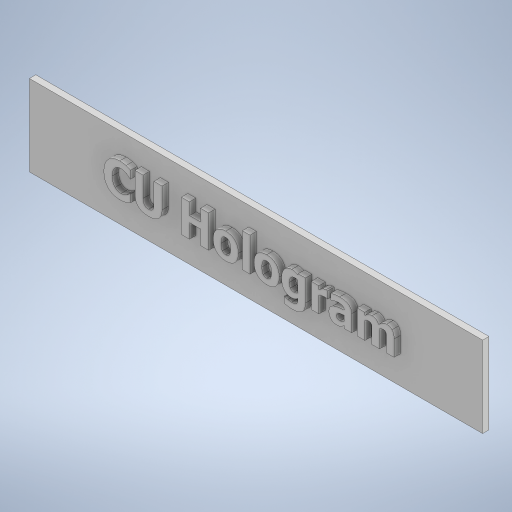
# Autodesk Inventor part: Apple iPad 2022 Hologram
Saved by Autodesk Inventor 2024 (Build 280153000, 153)
## iProperties
Created: 2024-02-23
Part Number: Apple iPad 2022 Hologram
Material: Generic
Document SubType Name: Modeling
Designer: littl
Density: 1 g/cm^3
Appearance: Default
Author: littl
Autodesk Inventor part; units mm, degrees
ref_plane "YZ Plane" through (0, 0, 0) normal (1, 0, 0) x (0, 1, 0)
ref_plane "Work Plane4" through (-177.8, 25.4, 133.35) normal (0, 0, 1) x (1, 0, 0)
sketch "Sketch7" plane through (-177.8, 25.4, 133.35) normal (0, 0, 1) x (1, 0, 0)
  line L0 (355.6, 0) -> (355.6, 12.7)
  line L1 (355.6, 12.7) -> (0, 12.7)
  line L2 (0, 12.7) -> (0, 0)
  line L3 (50.8, -25.4) -> (304.8, -25.4) projected
  line L4 (50.8, -25.4) -> (304.8, -25.4)
  line L5 (304.8, -50.8) -> (50.8, -50.8)
  line L6 (0, 12.7) -> (355.6, 12.7)
  line L7 (355.6, 12.7) -> (355.6, -50.8)
  line L8 (355.6, -50.8) -> (0, -50.8)
  line L9 (0, -50.8) -> (0, 12.7)
  point P0 (177.8, -25.4)
  point P1 (50.8, -50.8)
  dimension "d36" = 12.7
  dimension "d37" = 25.4
  constraints: 18 end point, 5 equal length, 1 horizontal, 1 perpendicular, 1 point on line
  measures "d36" distance of L0.end L0.start
  measures "d37" distance of L3.end L5.start
extrude "Decoration Plate" add sketch "Sketch7" along normal blind 5
ref_plane "Work Plane3" through (-177.8, 25.4, 138.35) normal (0, 0, 1) x (1, 0, 0)
sketch "Sketch8" plane through (-177.8, 25.4, 138.35) normal (0, 0, 1) x (1, 0, 0)
  line L0 (0, 12.7) -> (355.6, 12.7) construction
  line L1 (355.6, 12.7) -> (355.6, -50.8) construction
  line L2 (355.6, -50.8) -> (0, -50.8) construction
  line L3 (0, -50.8) -> (0, 12.7) construction
  line L4 (355.6, -50.8) -> (355.6, 12.7) projected
  line L5 (0, 12.7) -> (0, -50.8) projected
  line L6 (355.6, 12.7) -> (0, 12.7) projected
  line L7 (0, -50.8) -> (355.6, -50.8) projected
  spline S0 degree 2 poles (75.8604, -29.2079) (70.1382, -29.2079) (63.428, -22.2919) (63.428, -16.0345) knots 0 0 0 1 2 2 2
  spline S1 degree 2 poles (63.428, -16.0345) (63.428, -10.0036) (70.1588, -2.8199) (75.881, -2.8199) knots 0 0 0 1 2 2 2
  spline S2 degree 2 poles (75.881, -2.8199) (77.3836, -2.8199) (79.8124, -3.1699) (80.9239, -3.458) knots 0 0 0 1 2 2 2
  spline S3 degree 2 poles (80.9239, -3.458) (81.7884, -3.7256) (83.8262, -4.6107) (84.4643, -4.94) knots 0 0 0 1 2 2 2
  line L8 (84.4643, -4.94) -> (84.4643, -10.9916)
  line L9 (84.4643, -10.9916) -> (83.8262, -10.9916)
  spline S4 degree 2 poles (83.8262, -10.9916) (83.3528, -10.5799) (81.9531, -9.4272) (81.068, -8.8921) knots 0 0 0 1 2 2 2
  spline S5 degree 2 poles (81.068, -8.8921) (80.1829, -8.3363) (78.0628, -7.5747) (76.8896, -7.5747) knots 0 0 0 1 2 2 2
  spline S6 degree 2 poles (76.8896, -7.5747) (75.5105, -7.5747) (73.2257, -8.4392) (72.1759, -9.5301) knots 0 0 0 1 2 2 2
  spline S7 degree 2 poles (72.1759, -9.5301) (71.2291, -10.4976) (70.0147, -13.8115) (70.0147, -16.0551) knots 0 0 0 1 2 2 2
  spline S8 degree 2 poles (70.0147, -16.0551) (70.0147, -18.4222) (71.2703, -21.6538) (72.2994, -22.6418) knots 0 0 0 1 2 2 2
  spline S9 degree 2 poles (72.2994, -22.6418) (73.2874, -23.6092) (75.7163, -24.4532) (76.9307, -24.4532) knots 0 0 0 1 2 2 2
  spline S10 degree 2 poles (76.9307, -24.4532) (78.1863, -24.4532) (80.4711, -23.6092) (81.2532, -23.0947) knots 0 0 0 1 2 2 2
  spline S11 degree 2 poles (81.2532, -23.0947) (82.1178, -22.5801) (83.4145, -21.4891) (83.8879, -21.0569) knots 0 0 0 1 2 2 2
  line L10 (83.8879, -21.0569) -> (84.4643, -21.0569)
  line L11 (84.4643, -21.0569) -> (84.4643, -27.0261)
  spline S12 degree 2 poles (84.4643, -27.0261) (83.7644, -27.3554) (81.9325, -28.1788) (80.9445, -28.4669) knots 0 0 0 1 2 2 2
  spline S13 degree 2 poles (80.9445, -28.4669) (79.7507, -28.8374) (77.6717, -29.2079) (75.8604, -29.2079) knots 0 0 0 1 2 2 2
  spline S14 degree 2 poles (98.5022, -29.2491) (93.3769, -29.2491) (87.8605, -24.3091) (87.8605, -19.5337) knots 0 0 0 1 2 2 2
  line L12 (87.8605, -19.5337) -> (87.8605, -3.3139)
  line L13 (87.8605, -3.3139) -> (94.2414, -3.3139)
  line L14 (94.2414, -3.3139) -> (94.2414, -19.1632)
  spline S15 degree 2 poles (94.2414, -19.1632) (94.2414, -21.8185) (96.238, -24.412) (98.5022, -24.412) knots 0 0 0 1 2 2 2
  spline S16 degree 2 poles (98.5022, -24.412) (100.7046, -24.412) (102.763, -21.9214) (102.763, -19.1632) knots 0 0 0 1 2 2 2
  line L15 (102.763, -19.1632) -> (102.763, -3.3139)
  line L16 (102.763, -3.3139) -> (109.1438, -3.3139)
  line L17 (109.1438, -3.3139) -> (109.1438, -19.5131)
  spline S17 degree 2 poles (109.1438, -19.5131) (109.1438, -24.2062) (103.7716, -29.2491) (98.5022, -29.2491) knots 0 0 0 1 2 2 2
  line L18 (145.7001, -28.7139) -> (139.3192, -28.7139)
  line L19 (139.3192, -28.7139) -> (139.3192, -17.4548)
  line L20 (139.3192, -17.4548) -> (130.6536, -17.4548)
  line L21 (130.6536, -17.4548) -> (130.6536, -28.7139)
  line L22 (130.6536, -28.7139) -> (124.2727, -28.7139)
  line L23 (124.2727, -28.7139) -> (124.2727, -3.3139)
  line L24 (124.2727, -3.3139) -> (130.6536, -3.3139)
  line L25 (130.6536, -3.3139) -> (130.6536, -12.6177)
  line L26 (130.6536, -12.6177) -> (139.3192, -12.6177)
  line L27 (139.3192, -12.6177) -> (139.3192, -3.3139)
  line L28 (139.3192, -3.3139) -> (145.7001, -3.3139)
  line L29 (145.7001, -3.3139) -> (145.7001, -28.7139)
  spline S18 degree 2 poles (169.0006, -19.1426) (169.0006, -23.8768) (163.8341, -29.3109) (159.1205, -29.3109) knots 0 0 0 1 2 2 2
  spline S19 degree 2 poles (159.1205, -29.3109) (154.4275, -29.3109) (149.2199, -23.8768) (149.2199, -19.1426) knots 0 0 0 1 2 2 2
  spline S20 degree 2 poles (149.2199, -19.1426) (149.2199, -14.3673) (154.4275, -8.9538) (159.1205, -8.9538) knots 0 0 0 1 2 2 2
  spline S21 degree 2 poles (159.1205, -8.9538) (163.8135, -8.9538) (169.0006, -14.3878) (169.0006, -19.1426) knots 0 0 0 1 2 2 2
  spline S22 degree 2 poles (162.8873, -19.1838) (162.8873, -17.4754) (162.3315, -15.1906) (161.8375, -14.5113) knots 0 0 0 1 2 2 2
  spline S23 degree 2 poles (161.8375, -14.5113) (161.3024, -13.7909) (159.9644, -13.2352) (159.1205, -13.2352) knots 0 0 0 1 2 2 2
  spline S24 degree 2 poles (159.1205, -13.2352) (158.2972, -13.2352) (157.0004, -13.7292) (156.4652, -14.429) knots 0 0 0 1 2 2 2
  spline S25 degree 2 poles (156.4652, -14.429) (155.9507, -15.0877) (155.3331, -17.4136) (155.3331, -19.1838) knots 0 0 0 1 2 2 2
  spline S26 degree 2 poles (155.3331, -19.1838) (155.3331, -20.9334) (155.9095, -23.0947) (156.3829, -23.7533) knots 0 0 0 1 2 2 2
  spline S27 degree 2 poles (156.3829, -23.7533) (156.8563, -24.412) (158.2972, -25.0295) (159.1617, -25.0295) knots 0 0 0 1 2 2 2
  spline S28 degree 2 poles (159.1617, -25.0295) (159.8821, -25.0295) (161.3641, -24.412) (161.8169, -23.7945) knots 0 0 0 1 2 2 2
  spline S29 degree 2 poles (161.8169, -23.7945) (162.3315, -23.0741) (162.8873, -20.9951) (162.8873, -19.1838) knots 0 0 0 1 2 2 2
  line L30 (178.1396, -28.7139) -> (172.1704, -28.7139)
  line L31 (172.1704, -28.7139) -> (172.1704, -2.1818)
  line L32 (172.1704, -2.1818) -> (178.1396, -2.1818)
  line L33 (178.1396, -2.1818) -> (178.1396, -28.7139)
  spline S30 degree 2 poles (201.0902, -19.1426) (201.0902, -23.8768) (195.9237, -29.3109) (191.2101, -29.3109) knots 0 0 0 1 2 2 2
  spline S31 degree 2 poles (191.2101, -29.3109) (186.5171, -29.3109) (181.3095, -23.8768) (181.3095, -19.1426) knots 0 0 0 1 2 2 2
  spline S32 degree 2 poles (181.3095, -19.1426) (181.3095, -14.3673) (186.5171, -8.9538) (191.2101, -8.9538) knots 0 0 0 1 2 2 2
  spline S33 degree 2 poles (191.2101, -8.9538) (195.9032, -8.9538) (201.0902, -14.3878) (201.0902, -19.1426) knots 0 0 0 1 2 2 2
  spline S34 degree 2 poles (194.9769, -19.1838) (194.9769, -17.4754) (194.4212, -15.1906) (193.9272, -14.5113) knots 0 0 0 1 2 2 2
  spline S35 degree 2 poles (193.9272, -14.5113) (193.392, -13.7909) (192.0541, -13.2352) (191.2101, -13.2352) knots 0 0 0 1 2 2 2
  spline S36 degree 2 poles (191.2101, -13.2352) (190.3868, -13.2352) (189.09, -13.7292) (188.5549, -14.429) knots 0 0 0 1 2 2 2
  spline S37 degree 2 poles (188.5549, -14.429) (188.0403, -15.0877) (187.4228, -17.4136) (187.4228, -19.1838) knots 0 0 0 1 2 2 2
  spline S38 degree 2 poles (187.4228, -19.1838) (187.4228, -20.9334) (187.9991, -23.0947) (188.4725, -23.7533) knots 0 0 0 1 2 2 2
  spline S39 degree 2 poles (188.4725, -23.7533) (188.946, -24.412) (190.3868, -25.0295) (191.2513, -25.0295) knots 0 0 0 1 2 2 2
  spline S40 degree 2 poles (191.2513, -25.0295) (191.9717, -25.0295) (193.4537, -24.412) (193.9066, -23.7945) knots 0 0 0 1 2 2 2
  spline S41 degree 2 poles (193.9066, -23.7945) (194.4212, -23.0741) (194.9769, -20.9951) (194.9769, -19.1838) knots 0 0 0 1 2 2 2
  spline S42 degree 2 poles (221.6737, -26.5115) (221.6737, -29.1668) (220.1299, -32.8924) (218.8126, -33.9216) knots 0 0 0 1 2 2 2
  spline S43 degree 2 poles (218.8126, -33.9216) (217.4746, -34.9713) (213.7696, -35.9182) (211.5054, -35.9182) knots 0 0 0 1 2 2 2
  spline S44 degree 2 poles (211.5054, -35.9182) (209.5912, -35.9182) (206.1537, -35.4241) (204.8981, -35.0948) knots 0 0 0 1 2 2 2
  line L34 (204.8981, -35.0948) -> (204.8981, -30.2989)
  line L35 (204.8981, -30.2989) -> (205.598, -30.2989)
  spline S45 degree 2 poles (205.598, -30.2989) (206.0302, -30.4635) (207.2447, -30.8752) (207.8622, -31.0399) knots 0 0 0 1 2 2 2
  spline S46 degree 2 poles (207.8622, -31.0399) (208.6032, -31.2251) (210.0028, -31.4721) (210.7233, -31.4721) knots 0 0 0 1 2 2 2
  spline S47 degree 2 poles (210.7233, -31.4721) (212.2464, -31.4721) (214.2636, -30.8546) (214.7782, -30.2783) knots 0 0 0 1 2 2 2
  spline S48 degree 2 poles (214.7782, -30.2783) (215.2928, -29.6814) (215.7045, -28.0759) (215.7045, -26.8408) knots 0 0 0 1 2 2 2
  line L36 (215.7045, -26.8408) -> (215.7045, -26.4909)
  spline S49 degree 2 poles (215.7045, -26.4909) (214.6959, -27.376) (212.0612, -28.4464) (210.6615, -28.4464) knots 0 0 0 1 2 2 2
  spline S50 degree 2 poles (210.6615, -28.4464) (206.9359, -28.4464) (202.9015, -23.6092) (202.9015, -18.6486) knots 0 0 0 1 2 2 2
  spline S51 degree 2 poles (202.9015, -18.6486) (202.9015, -16.405) (204.1366, -12.8235) (205.2481, -11.5679) knots 0 0 0 1 2 2 2
  spline S52 degree 2 poles (205.2481, -11.5679) (206.3184, -10.3535) (209.303, -9.0361) (210.9291, -9.0361) knots 0 0 0 1 2 2 2
  spline S53 degree 2 poles (210.9291, -9.0361) (212.3905, -9.0361) (214.7165, -9.7771) (215.6633, -10.3947) knots 0 0 0 1 2 2 2
  line L37 (215.6633, -10.3947) -> (215.8897, -9.5507)
  line L38 (215.8897, -9.5507) -> (221.6737, -9.5507)
  line L39 (221.6737, -9.5507) -> (221.6737, -26.5115)
  line L40 (215.7045, -22.683) -> (215.7045, -13.9968)
  spline S54 degree 2 poles (215.7045, -13.9968) (215.2722, -13.7909) (213.9754, -13.5233) (213.3168, -13.5233) knots 0 0 0 1 2 2 2
  spline S55 degree 2 poles (213.3168, -13.5233) (211.1761, -13.5233) (209.0148, -16.3021) (209.0148, -18.7927) knots 0 0 0 1 2 2 2
  spline S56 degree 2 poles (209.0148, -18.7927) (209.0148, -20.0277) (209.3442, -21.7567) (209.7764, -22.4154) knots 0 0 0 1 2 2 2
  spline S57 degree 2 poles (209.7764, -22.4154) (210.2087, -23.0741) (211.5878, -23.7327) (212.6581, -23.7327) knots 0 0 0 1 2 2 2
  spline S58 degree 2 poles (212.6581, -23.7327) (213.4609, -23.7327) (215.0046, -23.177) (215.7045, -22.683) knots 0 0 0 1 2 2 2
  line L41 (239.1079, -15.2112) -> (238.6139, -15.2112)
  spline S59 degree 2 poles (238.6139, -15.2112) (238.2639, -15.0877) (236.9672, -14.9642) (236.185, -14.9642) knots 0 0 0 1 2 2 2
  spline S60 degree 2 poles (236.185, -14.9642) (235.2588, -14.9642) (233.1798, -15.5199) (232.2124, -15.8904) knots 0 0 0 1 2 2 2
  line L42 (232.2124, -15.8904) -> (232.2124, -28.7139)
  line L43 (232.2124, -28.7139) -> (226.2432, -28.7139)
  line L44 (226.2432, -28.7139) -> (226.2432, -9.5507)
  line L45 (226.2432, -9.5507) -> (232.2124, -9.5507)
  line L46 (232.2124, -9.5507) -> (232.2124, -12.3089)
  spline S61 degree 2 poles (232.2124, -12.3089) (232.6241, -11.9384) (234.0649, -10.7857) (234.6618, -10.4358) knots 0 0 0 1 2 2 2
  spline S62 degree 2 poles (234.6618, -10.4358) (235.3205, -10.0447) (237.0495, -9.489) (237.8111, -9.489) knots 0 0 0 1 2 2 2
  spline S63 degree 2 poles (237.8111, -9.489) (238.0993, -9.489) (238.8197, -9.5301) (239.1079, -9.5507) knots 0 0 0 1 2 2 2
  line L47 (239.1079, -9.5507) -> (239.1079, -15.2112)
  spline S64 degree 2 poles (251.9519, -26.6762) (251.3344, -27.1908) (250.367, -28.0141) (249.5437, -28.4258) knots 0 0 0 1 2 2 2
  spline S65 degree 2 poles (249.5437, -28.4258) (248.7409, -28.8169) (247.2177, -29.2285) (245.8592, -29.2285) knots 0 0 0 1 2 2 2
  spline S66 degree 2 poles (245.8592, -29.2285) (243.3069, -29.2285) (239.9518, -25.8117) (239.9518, -23.2182) knots 0 0 0 1 2 2 2
  spline S67 degree 2 poles (239.9518, -23.2182) (239.9518, -21.0981) (241.6602, -18.4634) (243.2657, -17.7018) knots 0 0 0 1 2 2 2
  spline S68 degree 2 poles (243.2657, -17.7018) (244.8918, -16.9196) (249.3996, -16.3021) (251.9931, -16.1374) knots 0 0 0 1 2 2 2
  line L48 (251.9931, -16.1374) -> (251.9931, -16.0345)
  spline S69 degree 2 poles (251.9931, -16.0345) (251.9931, -14.4496) (249.6466, -13.2352) (247.3001, -13.2352) knots 0 0 0 1 2 2 2
  spline S70 degree 2 poles (247.3001, -13.2352) (246.2503, -13.2352) (243.4098, -13.9968) (242.0719, -14.5937) knots 0 0 0 1 2 2 2
  line L49 (242.0719, -14.5937) -> (241.5573, -14.5937)
  line L50 (241.5573, -14.5937) -> (241.5573, -9.9624)
  spline S71 degree 2 poles (241.5573, -9.9624) (242.4424, -9.7154) (246.3944, -9.0156) (248.4116, -9.0156) knots 0 0 0 1 2 2 2
  spline S72 degree 2 poles (248.4116, -9.0156) (253.3516, -9.0156) (257.88, -12.3089) (257.88, -15.6846) knots 0 0 0 1 2 2 2
  line L51 (257.88, -15.6846) -> (257.88, -28.7139)
  line L52 (257.88, -28.7139) -> (251.9519, -28.7139)
  line L53 (251.9519, -28.7139) -> (251.9519, -26.6762)
  line L54 (251.9519, -23.7122) -> (251.9519, -19.7395)
  spline S73 degree 2 poles (251.9519, -19.7395) (250.4288, -19.8836) (248.5557, -20.11) (247.65, -20.4394) knots 0 0 0 1 2 2 2
  spline S74 degree 2 poles (247.65, -20.4394) (246.8472, -20.707) (245.9827, -21.8185) (245.9827, -22.7241) knots 0 0 0 1 2 2 2
  spline S75 degree 2 poles (245.9827, -22.7241) (245.9827, -24.0621) (247.4442, -25.0707) (248.8644, -25.0707) knots 0 0 0 1 2 2 2
  spline S76 degree 2 poles (248.8644, -25.0707) (249.6466, -25.0707) (251.2933, -24.3502) (251.9519, -23.7122) knots 0 0 0 1 2 2 2
  line L55 (285.1737, -28.7139) -> (285.1737, -19.1426)
  spline S77 degree 2 poles (285.1737, -19.1426) (285.1737, -17.7224) (285.0707, -15.7875) (284.8237, -15.17) knots 0 0 0 1 2 2 2
  spline S78 degree 2 poles (284.8237, -15.17) (284.5562, -14.5525) (283.4858, -13.9968) (282.5184, -13.9968) knots 0 0 0 1 2 2 2
  spline S79 degree 2 poles (282.5184, -13.9968) (281.8391, -13.9968) (280.5218, -14.5937) (279.7396, -15.1494) knots 0 0 0 1 2 2 2
  line L56 (279.7396, -15.1494) -> (279.7396, -28.7139)
  line L57 (279.7396, -28.7139) -> (273.7293, -28.7139)
  line L58 (273.7293, -28.7139) -> (273.7293, -19.1426)
  spline S80 degree 2 poles (273.7293, -19.1426) (273.7293, -17.7429) (273.6058, -15.7875) (273.3588, -15.17) knots 0 0 0 1 2 2 2
  spline S81 degree 2 poles (273.3588, -15.17) (273.0912, -14.5525) (272.0208, -13.9968) (271.0534, -13.9968) knots 0 0 0 1 2 2 2
  spline S82 degree 2 poles (271.0534, -13.9968) (270.333, -13.9968) (268.9127, -14.676) (268.2541, -15.1494) knots 0 0 0 1 2 2 2
  line L59 (268.2541, -15.1494) -> (268.2541, -28.7139)
  line L60 (268.2541, -28.7139) -> (262.2848, -28.7139)
  line L61 (262.2848, -28.7139) -> (262.2848, -9.5507)
  line L62 (262.2848, -9.5507) -> (268.2541, -9.5507)
  line L63 (268.2541, -9.5507) -> (268.2541, -11.6708)
  spline S83 degree 2 poles (268.2541, -11.6708) (269.7155, -10.4358) (272.3296, -9.0361) (273.9557, -9.0361) knots 0 0 0 1 2 2 2
  spline S84 degree 2 poles (273.9557, -9.0361) (275.7053, -9.0361) (278.3811, -10.7034) (279.081, -12.3707) knots 0 0 0 1 2 2 2
  spline S85 degree 2 poles (279.081, -12.3707) (280.7894, -10.7652) (283.8357, -9.0361) (285.4001, -9.0361) knots 0 0 0 1 2 2 2
  spline S86 degree 2 poles (285.4001, -9.0361) (286.738, -9.0361) (288.8581, -9.8801) (289.5785, -10.7446) knots 0 0 0 1 2 2 2
  spline S87 degree 2 poles (289.5785, -10.7446) (290.3813, -11.6708) (291.184, -14.2026) (291.184, -16.2404) knots 0 0 0 1 2 2 2
  line L64 (291.184, -16.2404) -> (291.184, -28.7139)
  line L65 (291.184, -28.7139) -> (285.1737, -28.7139)
  point P0 (177.8, -25.4)
  point P1 (355.6, -19.05)
  point P2 (355.6, -19.05)
  dimension "d40" = 0
  dimension "d41" = 0
  dimension "d42" = 0
  dimension "d43" = 0
  constraints: 2 midpoint, 2 other
  measures "d40" distance of point (355.6, -19.05) point (355.6, -19.05)
  measures "d41" distance between parallel lines of L5 L3
  measures "d42" distance between parallel lines of L6 L0
  measures "d43" distance between parallel lines of L7 L2
extrude "Decoration Text" add sketch "Sketch8" along normal blind 5 contours S0 S1 S2 S3 L8 L9 S4 S5 S6 S7 S8 S9 S10 S11 L10 L11 S12 S13 | S14 L12 L13 L14 S15 S16 L15 L16 L17 S17 | L18 L19 L20 L21 L22 L23 L24 L25 L26 L27 L28 L29 | S18 S19 S20 S21 | L30 L31 L32 L33 | S30 S31 S32 S33 | S42 S43 S44 L34 L35 S45 S46 S47 S48 L36 S49 S50 S51 S52 S53 L37 L38 L39 | L41 S59 S60 L42 L43 L44 L45 L46 S61 S62 S63 L47 | S64 S65 S66 S67 S68 L48 S69 S70 L49 L50 S71 S72 L51 L52 L53 | L55 S77 S78 S79 L56 L57 L58 S80 S81 S82 L59 L60 L61 L62 L63 S83 S84 S85 S86 S87 L64 L65
body "Solid1"
